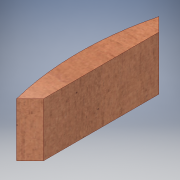
# Autodesk Inventor part: Short
Saved by Autodesk Inventor 2019 (Build 230136000, 136)
## iProperties
Created: 2019-05-01
Part Number: Short
Material: Красное дерево
Document SubType Name: Modeling
Designer: stepa
Density: 0.512 g/cm^3
Appearance: Красное дерево — натуральный — полированный
Author: stepa
Autodesk Inventor part; units mm, degrees
ref_plane "YZ Plane" through (0, 0, 0) normal (1, 0, 0) x (0, 1, 0)
ref_plane "XZ Plane" through (0, 0, 0) normal (0, 1, 0) x (-1, 0, 0)
ref_plane "XY Plane" through (0, 0, 0) normal (0, 0, 1) x (1, 0, 0)
sketch "Эскиз1" plane through (0, 0, 0) normal (1, 0, 0) x (0, 1, 0)
  line L0 (0, 0) -> (60, 0)
  line L1 (60, 0) -> (60, -178.77)
  line L2 (60, -178.77) -> (0, -178.77)
  line L3 (0, -178.77) -> (0, 0)
  dimension "d0" = 60
  dimension "d1" = 178.77
  constraints: 8 end point, 2 parallel, 1 horizontal, 1 perpendicular
  measures "d0" distance of L1.end L2.end
  measures "d1" distance of L0.end L1.end
extrude "Выдавливание1" add sketch "Эскиз1" along normal blind 25
chamfer "Фаска1" distance 25 angle 45 2 edges at (25, 30, 0) (25, 30, -178.77)
sketch "Эскиз2" plane through (0, 60, 0) normal (0, 1, 0) x (1, 0, 0)
  line L0 (25, 153.77) -> (3.5, 175.27) projected
  arc A0 (10, 168.77) -> (10, 10) centre (320.0989, 89.385) ccw
  line L1 (0, 0) -> (0, 178.77) projected
  line L2 (0, 89.385) -> (124.8295, 89.385)
  line L3 (25, 25) -> (0, 0) projected
  arc A1 (25, 153.77) -> (25, 25) centre (320.0989, 89.385) ccw
  line L4 (0, 178.77) -> (25, 153.77) projected
  line L5 (0, 0) -> (0, 178.77) projected
  line L6 (25, 25) -> (0, 0) projected
  line L7 (25, 153.77) -> (25, 25) projected
  line L8 (10, 10) -> (0, 0)
  line L9 (0, 0) -> (0, 89.385)
  line L10 (0, 89.385) -> (0, 178.77)
  line L11 (10, 168.77) -> (0, 178.77)
  line L12 (25, 153.77) -> (25, 25)
  point P0 (7, 178.77)
  dimension "d7" = 10
  constraints: 12 end point, 5 point on circle, 3 collinear, 2 centre point, 2 midpoint, 2 point on line, 2 tangent, 1 concentric, 1 horizontal, 1 parallel, 1 perpendicular, 2 other
  measures "d7" distance from line of L1 L8.start
extrude "Выдавливание2" cut sketch "Эскиз2" against normal blind 60 contours A0 L1 L4 L0 | A0 L3 L1
